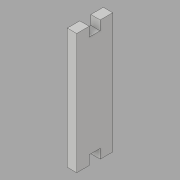
# Autodesk Inventor part: g_arm3
Saved by Autodesk Inventor 2019 (Build 230136000, 136)
## iProperties
Created: 2021-11-01
Part Number: g_arm3
Material: Generic
Document SubType Name: Modeling
Designer: Mohamed
Density: 1 g/cm^3
Appearance: Default
Author: Mohamed
Autodesk Inventor part; units mm, degrees
ref_plane "YZ Plane" through (0, 0, 0) normal (1, 0, 0) x (0, 1, 0)
ref_plane "XZ Plane" through (0, 0, 0) normal (0, 1, 0) x (-1, 0, 0)
ref_plane "XY Plane" through (0, 0, 0) normal (0, 0, 1) x (1, 0, 0)
sketch "Sketch1" plane through (0, 0, 0) normal (1, 0, 0) x (0, 1, 0)
  line L0 (0, 0) -> (77, 0)
  line L1 (77, 0) -> (77, -23)
  line L2 (77, -23) -> (0, -23)
  line L3 (0, -23) -> (0, 0)
  line L4 (71, -11.5) -> (71, -8)
  line L5 (71, -8) -> (71, -15)
  line L6 (71, -15) -> (77, -15)
  line L7 (71, -8) -> (77, -8)
  line L8 (0, -8) -> (6, -8)
  line L9 (6, -8) -> (6, -15)
  line L10 (6, -15) -> (0, -15)
  dimension "d0" = 77
  dimension "d1" = 23
  dimension "d3" = 3.5
  dimension "d4" = 7
  dimension "d5" = 6
  dimension "d6" = 7
  constraints: 22 end point, 5 point on line, 4 perpendicular, 3 parallel, 2 horizontal
  measures "d0" distance of L1.end L2.end
  measures "d1" distance of L0.end L1.end
  measures "d3" distance of L4.start L4.end
  measures "d4" distance of L4.end L5.end
  measures "d5" distance of L8.start L8.end
  measures "d6" distance of L8.end L9.end
extrude "Extrusion1" add sketch "Sketch1" along normal blind 6 contours L0 L1 L7 L4 L5 L6 L2 L3 L10 L9 L8
body "Solid1"
